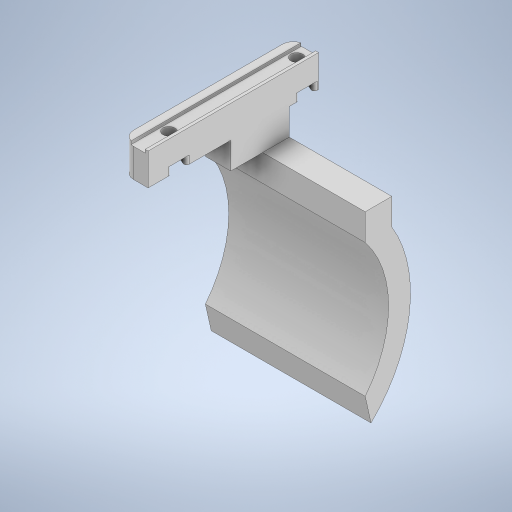
# Autodesk Inventor part: Back
Saved by Autodesk Inventor 2024 (Build 280153000, 153)
## iProperties
Created: 2023-12-18
Part Number: Back
Material: Generic
Document SubType Name: Modeling
Designer: Mechatronics Lab 1
Density: 1 g/cm^3
Appearance: Default
Author: Mechatronics Lab 1
Autodesk Inventor part; units mm, degrees
ref_plane "YZ Plane" through (0, 0, 0) normal (1, 0, 0) x (0, 1, 0)
ref_plane "XZ Plane" through (0, 0, 0) normal (0, 1, 0) x (-1, 0, 0)
ref_plane "XY Plane" through (0, 0, 0) normal (0, 0, 1) x (1, 0, 0)
sketch "Sketch1" plane through (0, 0, 0) normal (0, 1, 0) x (-1, 0, 0)
  line L0 (0, 0) -> (9.5, 0)
  line L1 (9.5, 0) -> (9.5, -64)
  line L2 (9.5, -64) -> (0, -64)
  line L3 (0, -64) -> (0, 0)
  circle A0 centre (3.7, -11.5) radius 2.25
  circle A1 centre (3.7, -59.5) radius 2.25
  line L4 (3.7, -11.5) -> (3.7, -59.5) construction
  dimension "d1" = 9.5
  dimension "d2" = 64
  dimension "d3" = 4.5
  dimension "d4" = 48
  dimension "d6" = 3.7
  dimension "d17" = 4.5
  constraints: 10 end point, 2 centre point, 2 parallel, 1 equal radius, 1 horizontal, 1 perpendicular, 1 vertical
  measures "d1" distance of L0.start L0.end
  measures "d2" distance of L0.end L1.end
  measures "d3" diameter of A0
  measures "d4" distance of L4.start L4.end
  measures "d6" distance between parallel lines of L3 L4
  measures "d17" distance from line of L4.end L2
extrude "Extrusion1" add sketch "Sketch1" along normal blind 12
sketch "Sketch2" plane through (-9.5, 0, 0) normal (0, 0, 1) x (1, 0, 0)
  line L0 (9.5, 12) -> (0, 12) projected
  line L1 (3, 12) -> (8.4, 12)
  line L2 (8.4, 12) -> (8.4, 10.8)
  line L3 (8.4, 10.8) -> (3, 10.8)
  line L4 (3, 10.8) -> (3, 12)
  line L5 (9.5, 0) -> (9.5, 12) projected
  line L6 (3.55, 0) -> (8.05, 0) projected
  line L7 (3.55, 12) -> (8.05, 12) projected
  line L8 (9.5, 0) -> (9.5, 12) projected
  line L9 (9.5, 0) -> (9.5, 12) projected
  line L10 (3.55, 12) -> (8.05, 12) projected
  line L11 (3.55, 12) -> (3.55, 0) projected
  line L12 (3.55, 12) -> (8.05, 12) projected
  line L13 (3.55, 0) -> (8.05, 0) projected
  line L14 (3.55, 12) -> (8.05, 12) projected
  line L15 (3.55, 0) -> (8.05, 0) projected
  line L16 (3.55, 12) -> (8.05, 12) projected
  line L17 (3.55, 0) -> (8.05, 0) projected
  dimension "d9" = 1.1
  dimension "d10" = 5.4
  dimension "d11" = 1.2
  dimension "d76" = 12
  constraints: 8 end point, 2 parallel, 1 horizontal, 1 perpendicular, 1 point on line
  measures "d9" distance between parallel lines of L5 L2
  measures "d10" distance of L2.end L3.end
  measures "d11" distance between parallel lines of L0 L3
  measures "d76" distance between parallel lines of L6 L7
extrude "Extrusion2" cut sketch "Sketch2" against normal up to next
sketch "Sketch3" plane through (0, 0, 0) normal (0, -1, 0) x (1, 0, 0)
  circle A0 centre (-3.7, -11.5) radius 2.25 projected
  circle A1 centre (-3.7, -11.5) radius 3.75
  circle A2 centre (-3.7, -59.5) radius 2.25 projected
  circle A3 centre (-3.7, -59.5) radius 3.75
  point P0 (0, 0)
  dimension "d14" = 7.5
  constraints: 2 centre point, 2 coincident, 1 equal radius
  measures "d14" diameter of A3
extrude "Extrusion3" cut sketch "Sketch3" against normal blind 3
fillet "Fillet1" radius 1 4 edges at (0, 1.5, -58.8897) (0, 1.5, -60.1103) (0, 1.5, -10.8897) (0, 1.5, -12.1103)
fillet "Fillet2" radius 4 2 edges at (-9.5, 6, -64) (-9.5, 6, 0)
sketch "Sketch28" plane through (0, 0, 0) normal (0, -1, 0) x (1, 0, 0)
  arc A0 (-1.5684, -56.4147) -> (0, -55.592) centre (-1, -55.592) ccw projected
  line L0 (0, -55.592) -> (0, -53)
  line L1 (0, -15.408) -> (0, -55.592) projected
  line L2 (-9.5, -60) -> (-9.5, -4) projected
  line L3 (0, -53) -> (-9.5, -53)
  line L4 (-9.5, -53) -> (-9.5, -31)
  line L5 (-9.5, -31) -> (0, -31)
  line L6 (0, -31) -> (0, -53)
  point P0 (0, 0)
  point P1 (0, -31)
  dimension "d107" = 2.592
  dimension "d108" = 22
  constraints: 10 end point, 2 parallel, 2 point on line, 1 horizontal, 1 perpendicular
  measures "d107" distance of L0.start L0.end
  measures "d108" distance of L3.end L4.end
extrude "Extrusion19" add sketch "Sketch28" along normal blind 10
sketch "Sketch29" plane through (0, -10, 0) normal (0, -1, 0) x (1, 0, 0)
  line L0 (-9.5, -53) -> (0, -53) projected
  line L1 (-9.5, -53) -> (38.5, -53)
  line L2 (38.5, -53) -> (38.5, -43)
  line L3 (38.5, -43) -> (-21.5, -43)
  line L4 (-21.5, -43) -> (-21.5, -53)
  line L5 (-21.5, -53) -> (-9.5, -53)
  point P0 (0, 0)
  dimension "d111" = 48
  dimension "d112" = 10
  dimension "d113" = 60
  dimension "d114" = 10
  constraints: 10 end point, 2 perpendicular, 1 point on line, 1 vertical
  measures "d111" distance of L0.start L1.end
  measures "d112" distance of L1.end L2.end
  measures "d113" distance of L2.end L3.end
  measures "d114" distance of L3.end L4.end
extrude "Extrusion20" add sketch "Sketch29" along normal blind 10
sketch "Sketch30" plane through (-21.5, -10, -53) normal (-1, 0, 0) x (0, 0, 1)
  arc A0 (10, -10) -> (10, -60) centre (41.225, -35) ccw
  point P0 (53, 10)
  dimension "d117" = 50
  dimension "d118" = 40
  constraints: 2 point on circle, 1 centre point
  measures "d117" distance of A0.start A0.end
  measures "d118" radius of A0
sketch "Sketch31" plane through (0, -20, 0) normal (0, -1, 0) x (1, 0, 0)
  line L0 (-21.5, -43) -> (-21.5, -53) projected
  line L1 (38.5, -43) -> (-21.5, -43) projected
  line L2 (-21.5, -53) -> (38.5, -53)
  line L3 (38.5, -53) -> (38.5, -43)
  line L4 (38.5, -43) -> (-21.5, -43)
  line L5 (-21.5, -43) -> (-21.5, -53)
  point P0 (0, 0)
  constraints: 8 end point, 2 parallel, 1 horizontal, 1 perpendicular
sweep "Sweep1" add profiles "Sketch31" path "Sketch30"
body "Solid1"
